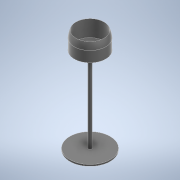
# Autodesk Inventor part: Magic 3D Sketch
Saved by Autodesk Inventor 2021 (Build 250183000, 183)
## iProperties
Created: 2021-07-29
Part Number: Magic 3D Sketch
Material: UHMW, Black
Document SubType Name: Modeling
Designer: Shammy Haider
Mass: 0.0155 g
Surface Area: 1.57478 cm^2
Volume: 0.0164894 cm^3
Density: 0.94 g/cm^3
Appearance: Smooth - Black
Author: Shammy Haider
Autodesk Inventor part; units mm, degrees
ref_plane "YZ Plane" through (0, 0, 0) normal (1, 0, 0) x (0, 1, 0)
ref_plane "XZ Plane" through (0, 0, 0) normal (0, 1, 0) x (-1, 0, 0)
ref_plane "XY Plane" through (0, 0, 0) normal (0, 0, 1) x (1, 0, 0)
sketch "Sketch1" plane through (0, 0, 0) normal (1, 0, 0) x (0, 1, 0)
  line L0 (13.9494, 0.6112) -> (11.5918, 0.6112)
  line L1 (11.5918, 0.6112) -> (10.3693, 2.5323)
  line L2 (10.3693, 2.5323) -> (0, 2.5323)
  line L3 (0, 2.5323) -> (0, 0)
  line L4 (13.9494, 0.8295) -> (11.7116, 0.8295)
  line L5 (11.7116, 0.8295) -> (10.4891, 2.7506)
  line L6 (10.4891, 2.7506) -> (-0.2183, 2.7506)
  line L7 (-0.2183, 2.7506) -> (-0.2183, 0)
  line L8 (13.9494, 0.8295) -> (13.9494, 0.6112)
  line L9 (0, 0) -> (-0.2183, 0)
  constraints: 20 end point, 4 perpendicular, 2 parallel, 1 horizontal, 3 other
revolve "Revolution1" add sketch "Sketch1" angle 360 about axis through (0, 10.4891, 2.7506) along (0, -1, 0)
fillet "Fillet1" radius 2 1 edges at (0, 13.9494, 4.8899)
body "Solid1"
